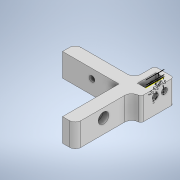
# Autodesk Inventor part: Vertical_1_v1
Saved by Autodesk Inventor 2020.3 (Build 243373000, 373)
## iProperties
Created: 2021-04-05
Part Number: Vertical_1_v1
Material: Generic
Document SubType Name: Modeling
Designer: sanyi
Density: 1 g/cm^3
Appearance: Default
Author: sanyi
Autodesk Inventor part; units mm, degrees
ref_plane "YZ Plane" through (0, 0, 0) normal (1, 0, 0) x (0, 1, 0)
ref_plane "XZ Plane" through (0, 0, 0) normal (0, 1, 0) x (-1, 0, 0)
ref_plane "XY Plane" through (0, 0, 0) normal (0, 0, 1) x (1, 0, 0)
sketch "Sketch1" plane through (0, 0, 0) normal (0, 1, 0) x (-1, 0, 0)
  line L0 (0, 0) -> (0, 40)
  line L1 (0, 40) -> (-9, 40)
  line L2 (-9, 40) -> (-9, 0)
  line L3 (-9, -9) -> (-1.8, -9) construction
  line L4 (40, -9) -> (40, 0)
  line L5 (40, 0) -> (0, 0)
  line L6 (0, 0) -> (-9, 0)
  line L7 (-15.4, 0) -> (-15.4, -23.5)
  line L8 (-15.4, -23.5) -> (-1.8, -23.5)
  line L9 (-1.8, -23.5) -> (-1.8, 0)
  line L10 (-11.9, -7) -> (-6.1, -7)
  line L11 (-6.1, -7) -> (-6.1, -20)
  line L12 (-6.1, -20) -> (-11.9, -20)
  line L13 (-11.9, -20) -> (-11.9, -7)
  line L14 (11.9662, -13.5) -> (-24.6607, -13.5) construction
  line L15 (-9, 12.1474) -> (-9, -36.694) construction
  line L16 (-1.8, -9) -> (40, -9)
  line L17 (-9, 0) -> (-9, -9) construction
  line L18 (-1.8, -9) -> (0, -9)
  arc A0 (-9, 0) -> (0, -9) centre (0, 0) ccw construction
  line L19 (-1.8, -1.8) -> (-15.4, -1.8) construction
  line L20 (-15.4, 0) -> (-9, 0)
  arc A1 (-1.8, -7.2) -> (-9, 0) centre (-9, -7.2) ccw
  point P0 (0, -9)
  dimension "d0" = 40
  dimension "d3" = 9
  dimension "d4" = 5.8
  dimension "d5" = 13
  dimension "d7" = 9
  dimension "d9" = 4.3
  dimension "d10" = 7
  dimension "d11" = 3.5
  dimension "d12" = 1.8
  dimension "d43" = 3.5
  constraints: 42 end point, 15 perpendicular, 9 point on line, 6 parallel, 4 point on circle, 3 horizontal, 3 tangent, 2 centre point, 1 collinear, 1 vertical, 2 other
  measures "d0" distance of L0.start L0.end
  measures "d3" distance of L0.end L1.end
  measures "d4" distance of L12.end L11.end
  measures "d5" distance of L11.end L10.end
  measures "d7" distance between parallel lines of L0 L15
  measures "d9" distance between parallel lines of L9 L11
  measures "d10" distance between parallel lines of L5 L10
  measures "d11" distance between parallel lines of L7 L13
  measures "d12" distance between parallel lines of L6 L19
  measures "d43" distance between parallel lines of L8 L12
extrude "Extrusion1" add sketch "Sketch1" along normal blind 16.4 contours L6 L2 L1 L0 | L5 L4 L16 L9 L6 | L9 A1 L6
extrude "Extrusion3" add sketch "Sketch1" along normal blind 16.4 contours A1 L9 L8 L7 L20
sketch "Sketch5" plane through (11.9, 0, -20) normal (-1, 0, 0) x (0, 0, 1)
  line L0 (0, 0) -> (0, 16.4) projected
  line L1 (0, 0) -> (13, 0) projected
  line L2 (13, 0) -> (13, 16.4) projected
  line L3 (13, 17) -> (0, 17)
  line L4 (11.1042, 11.4) -> (1.4974, 11.4) construction
  line L5 (13, 9.9) -> (0, 9.9)
  line L6 (13, 0) -> (13, 16.4) projected
  line L7 (13, 5.9) -> (0, 5.9)
  line L8 (0, 0) -> (0, 16.4) projected
  circle A0 centre (9.75, 11.4) radius 1
  circle A1 centre (3.25, 11.4) radius 1
  line L9 (6.5, 16.4) -> (6.5, 0) construction
  circle A2 centre (6.5, 5.9) radius 2.5
  line L10 (13, 5.9) -> (7.4615, 3.5923)
  line L11 (5.5385, 3.5923) -> (0, 5.9)
  line L12 (0, 16.4) -> (13, 16.4) projected
  line L13 (13, 18.2) -> (0, 18.2)
  line L14 (13, 21.4) -> (0, 21.4)
  point P0 (20, 0)
  dimension "d47" = 4
  dimension "d48" = 1.5
  dimension "d49" = 2
  dimension "d50" = 6.5
  dimension "d51" = 5.6
  dimension "d52" = 5
  dimension "d53" = 6.5
  dimension "d54" = 6.8
  dimension "d55" = 10
  constraints: 18 end point, 9 point on line, 3 centre point, 3 midpoint, 2 horizontal, 2 perpendicular, 2 point on circle, 2 tangent, 1 equal radius, 1 symmetric about line
  measures "d47" distance between parallel lines of L5 L7
  measures "d48" distance between parallel lines of L5 L4
  measures "d49" diameter of A0
  measures "d50" distance of A0.centre A1.centre
  measures "d51" distance between parallel lines of L3 L4
  measures "d52" diameter of A2
  measures "d53" distance between parallel lines of L12 L5
  measures "d54" distance between parallel lines of L13 L4
  measures "d55" distance between parallel lines of L14 L4
sketch "Sketch6" plane through (9, 0, 40) normal (1, 0, 0) x (0, 0, -1)
  line L0 (0, 0) -> (40, 0) projected
  line L1 (40, 0) -> (40, 16.4) projected
  line L2 (0, 16.4) -> (40, 16.4)
  line L3 (0, 0) -> (0, 16.4) projected
  line L4 (40, 16.4) -> (0, 16.4) projected
  line L5 (40, 16.4) -> (40, 0)
  line L6 (20, 22.8503) -> (20, -7.1359)
  line L7 (40, 0) -> (40, 16.4) projected
  line L8 (0, 16.4) -> (40, 16.4)
  line L9 (6.3453, 8.2) -> (32.3944, 8.2)
  circle A0 centre (20, 10) radius 3.75
  circle A1 centre (20, 10) radius 2
  dimension "d56" = 7.5
  dimension "d57" = 4
  dimension "d71" = 10
  constraints: 10 end point, 2 centre point, 1 coincident, 1 horizontal, 1 parallel, 1 perpendicular, 1 point on line, 2 other
  measures "d56" diameter of A0
  measures "d57" diameter of A1
  measures "d71" distance from line of L0 A0.centre
extrude "Extrusion7" cut sketch "Sketch6" against normal up to surface (9 mm away) contours A1 L9 L6 | L6 L9 A1 | L9 A1 L6 | L6 A1 L9
extrude "Extrusion8" cut sketch "Sketch6" against normal blind 4 contours A0 L9 A1 L6 | L6 A1 L9 A0 | A0 L6 A1 L9 | L9 A1 L6 A0
extrude "Extrusion9" add sketch "Sketch5" along normal up to surface (5.8 mm away) contours L0 L11 A2 L10 L2 L1
extrude "Extrusion10" cut sketch "Sketch5" along normal through all contours A2 L7 | L7 A2
sketch "Sketch8" plane through (-40, 0, -9) normal (0, 0, -1) x (-1, 0, 0)
  line L0 (-41.8, 0) -> (0, 0) projected
  line L1 (0, 0) -> (0, 16.4) projected
  line L2 (-41.8, 16.4) -> (0, 16.4)
  line L3 (-41.8, 0) -> (-41.8, 16.4)
  line L4 (-34.8875, 8.2) -> (-7.09, 8.2) construction
  line L5 (-20.9, 24.3165) -> (-20.9, -8.6206) construction
  circle A0 centre (-20.9, 10) radius 2
  circle A1 centre (-20.9, 10) radius 3.75
  point P0 (-40, 0)
  dimension "d69" = 4
  dimension "d70" = 7.5
  dimension "d72" = 10
  constraints: 8 end point, 3 parallel, 2 centre point, 1 coincident, 1 perpendicular, 1 point on line, 2 other
  measures "d69" diameter of A0
  measures "d70" diameter of A1
  measures "d72" distance from line of L0 A0.centre
extrude "Extrusion11" cut sketch "Sketch8" against normal up to surface (9 mm away) contours A0
extrude "Extrusion12" cut sketch "Sketch8" against normal blind 4 contours A1
fillet "Fillet4" radius 4 2 edges at (9, 8.2, 40) (-40, 8.2, -9)
fillet "Fillet4" radius 5 2 edges at (9, 8.2, 0) (1.8, 8.2, -9)
fillet "Fillet4" radius 2 3 edges at (15.4, 8.2, 0) (15.4, 8.2, -23.5) (1.8, 8.2, -23.5)
sketch "Sketch9" plane through (15.4, 0, -1.9742) normal (1, 0, 0) x (0, 0, -1)
  circle A0 centre (8.2758, 11.4) radius 1 projected
  circle A1 centre (14.7758, 11.4) radius 1 projected
  circle A2 centre (8.2758, 11.4) radius 2.15
  circle A3 centre (14.7758, 11.4) radius 2.15
  point P0 (-1.9742, 0)
  dimension "d80" = 4.3
  constraints: 2 centre point, 2 coincident, 1 equal radius
  measures "d80" diameter of A2
extrude "Extrusion13" cut sketch "Sketch9" against normal up to surface (3.5 mm away) contours A0 | A1
extrude "Extrusion14" cut sketch "Sketch9" against normal blind 2
ref_plane "Work Plane2" through (-3.2, 0, -21.5) normal (-1, 0, 0) x (0, 0, 1)
sketch "Sketch10" plane through (-3.2, 0, -21.5) normal (-1, 0, 0) x (0, 0, 1)
  circle A0 centre (4.75, 11.4) radius 1 projected
  circle A1 centre (11.25, 11.4) radius 1 projected
  circle A2 centre (4.75, 11.4) radius 1.5
  circle A3 centre (11.25, 11.4) radius 1.5
  circle A4 centre (4.75, 11.4) radius 2.5
  circle A5 centre (11.25, 11.4) radius 2.5
  point P0 (21.5, 0)
  dimension "d86" = 3
  dimension "d87" = 5
  constraints: 4 centre point, 3 coincident, 2 equal radius
  measures "d86" diameter of A2
  measures "d87" diameter of A4
extrude "Extrusion15" cut sketch "Sketch10" against normal blind 10 contours A0 | A1 | A2 | A3
extrude "Extrusion16" cut sketch "Sketch10" against normal blind 5.5 contours A4 | A5
body "Solid1"
